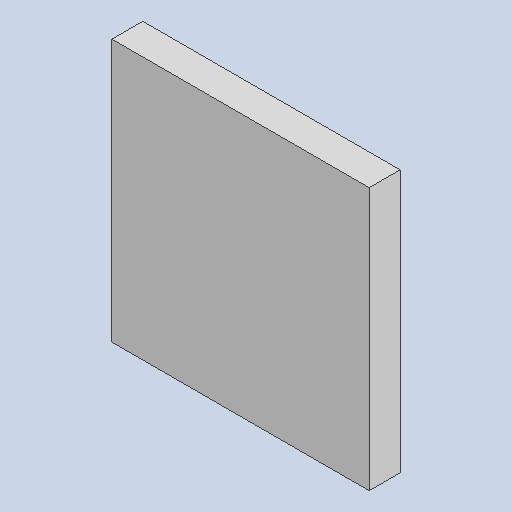
# Autodesk Inventor part: head_side
Saved by Autodesk Inventor 2024 (Build 280153000, 153)
## iProperties
Created: 2024-09-18
Part Number: head_side
Material: 일반
Document SubType Name: Modeling
Designer: Eungang
Density: 1 g/cm^3
Appearance: 기본값
Author: Eungang
Autodesk Inventor part; units mm, degrees
ref_plane "YZ Plane" through (0, 0, 0) normal (1, 0, 0) x (0, 1, 0)
ref_plane "XZ Plane" through (0, 0, 0) normal (0, 1, 0) x (-1, 0, 0)
ref_plane "XY Plane" through (0, 0, 0) normal (0, 0, 1) x (1, 0, 0)
sketch "스케치1" plane through (0, 0, 0) normal (0, 0, 1) x (1, 0, 0)
  line L0 (0, 0) -> (50, 0) projected
  line L1 (50, 0) -> (50, 25) projected
  line L2 (0, 25) -> (50, 25) projected
  line L3 (0, 0) -> (0, 25) projected
  line L4 (8.4, 0) -> (0, 0) projected
  line L5 (0, 0) -> (0, -16) projected
  line L6 (50, -16) -> (0, -16) projected
  line L7 (50, 0) -> (50, -16) projected
  line L8 (50, 0) -> (41.6, 0) projected
  line L9 (41.6, 0) -> (41.6, -10) projected
  line L10 (41.6, -10) -> (8.4, -10) projected
  line L11 (8.4, 0) -> (8.4, -10) projected
  line L12 (0, 25) -> (50, 25)
  line L13 (50, 25) -> (50, 35)
  line L14 (50, 35) -> (0, 35)
  line L15 (0, 35) -> (0, 25)
  line L16 (0, -16) -> (50, -16)
  line L17 (50, -16) -> (50, 35)
  line L18 (50, 35) -> (0, 35)
  line L19 (0, 35) -> (0, -16)
  dimension "d0" = 10
  constraints: 16 end point, 4 parallel, 2 horizontal, 2 perpendicular, 1 point on line
  measures "d0" distance of L13.end L12.end
extrude "돌출1" add sketch "스케치1" along normal blind 6
